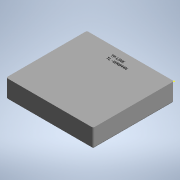
# Autodesk Inventor part: tplink nuevo
Saved by Autodesk Inventor 2022 (Build 260153000, 153)
## iProperties
Part Number: tplink nuevo
Material: Genérico
Document SubType Name: Modelado
Designer: andre
Appearance: Por defecto
Author: andre
Autodesk Inventor part; units mm, degrees
ref_plane "Plano YZ" through (0, 0, 0) normal (1, 0, 0) x (0, 1, 0)
ref_plane "Plano XZ" through (0, 0, 0) normal (0, 1, 0) x (-1, 0, 0)
ref_plane "Plano XY" through (0, 0, 0) normal (0, 0, 1) x (1, 0, 0)
sketch "Boceto1" plane through (0, 0, 0) normal (0, 1, 0) x (-1, 0, 0)
  line L0 (115, 106.7) -> (0, 106.7)
  line L1 (0, 106.7) -> (0, 0)
  line L2 (0, 0) -> (115, 0)
  line L3 (115, 0) -> (115, 106.7)
  dimension "d0" = 115
  dimension "d1" = 106.7
  constraints: 8 end point, 2 parallel, 1 horizontal, 1 perpendicular
  measures "d0" distance of L0.start L0.end
  measures "d1" distance of L2.end L0.start
extrude "Extrusión1" add sketch "Boceto1" along normal blind 24.3
fillet "Empalme1" radius 2 8 edges at (0, 12.15, 106.7) (0, 0, 53.35) (-57.5, 0, 106.7) (0, 12.15, 0) (-57.5, 0, 0) (-115, 12.15, 0) (-115, 0, 53.35) (-115, 12.15, 106.7)
sketch "Boceto2" plane through (0, 0, 0) normal (0, -1, 0) x (1, 0, 0)
  line L0 (-113, 104.7) -> (-2, 104.7) projected
  line L1 (-2, 104.7) -> (-2, 2) projected
  line L2 (-2, 104.7) -> (-2, 2) projected
  line L3 (-113, 104.7) -> (-2, 104.7) projected
  line L4 (-113, 2) -> (-113, 104.7) projected
  line L5 (-2, 2) -> (-113, 2) projected
  line L6 (-57.5, 104.7) -> (-57.5, 2) construction
  line L7 (-113, 106.7) -> (-2, 106.7) construction
  line L8 (-57.5, 53.35) -> (-57.5, 93.35) construction
  line L9 (-57.5, 93.35) -> (-57.5, 13.35) construction
  line L10 (-57.5, 93.35) -> (-50.5, 93.35) construction
  arc A0 (-50.5, 90.915) -> (-50.5, 95.785) centre (-50.5, 93.35) ccw construction
  line L11 (-57.5, 93.35) -> (-64.5, 93.35) construction
  arc A1 (-64.5, 95.785) -> (-64.5, 90.915) centre (-64.5, 93.35) ccw construction
  line L12 (-50.5, 90.915) -> (-52.9223, 90.915) construction
  line L13 (-50.5, 95.785) -> (-52.9223, 95.785) construction
  line L14 (-64.5, 95.785) -> (-62.0777, 95.785) construction
  line L15 (-64.5, 90.915) -> (-62.0777, 90.915) construction
  arc A2 (-64.5, 95.785) -> (-64.5, 90.915) centre (-64.5, 93.35) ccw
  arc A3 (-50.5, 90.915) -> (-50.5, 95.785) centre (-50.5, 93.35) ccw
  line L16 (-50.5, 90.915) -> (-52.9223, 90.915)
  line L17 (-50.5, 95.785) -> (-52.9223, 95.785)
  line L18 (-64.5, 95.785) -> (-62.0777, 95.785)
  line L19 (-64.5, 90.915) -> (-62.0777, 90.915)
  arc A4 (-62.0777, 90.915) -> (-52.9223, 90.915) centre (-57.5, 93.35) ccw construction
  arc A5 (-52.9223, 95.785) -> (-62.0777, 95.785) centre (-57.5, 93.35) ccw construction
  arc A6 (-62.0777, 90.915) -> (-52.9223, 90.915) centre (-57.5, 93.35) ccw
  arc A7 (-52.9223, 95.785) -> (-62.0777, 95.785) centre (-57.5, 93.35) ccw
  line L20 (-57.5, 53.35) -> (-46.2835, 53.35)
  line L21 (-46.2835, 53.35) -> (-72.4945, 53.35)
  line L22 (-57.5, 13.35) -> (-50.5, 13.35) construction
  arc A8 (-50.5, 10.915) -> (-50.5, 15.785) centre (-50.5, 13.35) ccw construction
  line L23 (-57.5, 13.35) -> (-64.5, 13.35) construction
  arc A9 (-64.5, 15.785) -> (-64.5, 10.915) centre (-64.5, 13.35) ccw construction
  line L24 (-50.5, 10.915) -> (-52.9223, 10.915) construction
  line L25 (-50.5, 15.785) -> (-52.9223, 15.785) construction
  line L26 (-64.5, 15.785) -> (-62.0777, 15.785) construction
  line L27 (-64.5, 10.915) -> (-62.0777, 10.915) construction
  arc A10 (-64.5, 15.785) -> (-64.5, 10.915) centre (-64.5, 13.35) ccw
  arc A11 (-50.5, 10.915) -> (-50.5, 15.785) centre (-50.5, 13.35) ccw
  line L28 (-50.5, 10.915) -> (-52.9223, 10.915)
  line L29 (-50.5, 15.785) -> (-52.9223, 15.785)
  line L30 (-64.5, 15.785) -> (-62.0777, 15.785)
  line L31 (-64.5, 10.915) -> (-62.0777, 10.915)
  arc A12 (-62.0777, 10.915) -> (-52.9223, 10.915) centre (-57.5, 13.35) ccw construction
  arc A13 (-52.9223, 15.785) -> (-62.0777, 15.785) centre (-57.5, 13.35) ccw construction
  arc A14 (-62.0777, 10.915) -> (-52.9223, 10.915) centre (-57.5, 13.35) ccw
  arc A15 (-52.9223, 15.785) -> (-62.0777, 15.785) centre (-57.5, 13.35) ccw
  point P0 (0, 0)
  dimension "d5" = 111
  dimension "d7" = 40
  dimension "d11" = 7
  dimension "d13" = 7
  dimension "d15" = 4.87
  dimension "d17" = 4.87
  dimension "d18" = 7
  dimension "d19" = 7
  dimension "d20" = 4.87
  dimension "d21" = 4.87
  constraints: 50 end point, 32 point on circle, 16 centre point, 12 coincident, 11 horizontal, 10 tangent, 6 equal length, 3 midpoint, 3 point on line, 1 perpendicular
  measures "d5" distance of L0.start L0.end
  measures "d7" distance of L8.start L8.end
  measures "d11" distance of L10.start L10.end
  measures "d13" distance of L10.start L11.end
  measures "d15" diameter of A2
  measures "d17" diameter of A3
  measures "d18" distance of L9.end L22.end
  measures "d19" distance of L9.end L23.end
  measures "d20" diameter of A10
  measures "d21" diameter of A11
extrude "Extrusión2" cut sketch "Boceto2" against normal blind 21 contours L18 A7 L17 A3 L16 A6 L19 A2 | L30 A15 L29 A11 L28 A14 L31 A10
sketch "Boceto4" plane through (0, 24.3, 0) normal (0, 1, 0) x (1, 0, 0)
  line L0 (-71.2801, -9.805) -> (-44.2711, -9.805) construction
  line L1 (-44.2711, -9.805) -> (-44.2711, -97.4462) construction
  line L2 (-44.2711, -97.4462) -> (-71.2801, -97.4462) construction
  line L3 (-71.2801, -97.4462) -> (-71.2801, -9.805) construction
  point P0 (0, 0)
  constraints: 2 other
